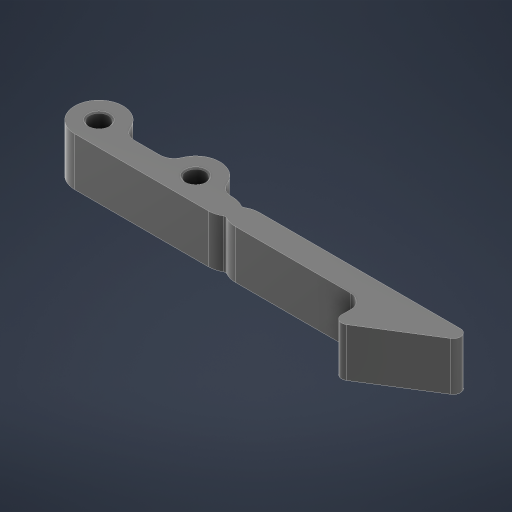
# Autodesk Inventor part: Battery_Clip
Saved by Autodesk Inventor 2024 (Build 280153000, 153)
## iProperties
Created: 2023-06-19
Part Number: Battery_Clip
Material: Nylon 6/6
Document SubType Name: Modeling
Designer: dzw04
Density: 1.13 g/cm^3
Appearance: Smooth - Black
Author: dzw04
Autodesk Inventor part; units mm, degrees
ref_plane "YZ Plane" through (0, 0, 0) normal (1, 0, 0) x (0, 1, 0)
ref_plane "XZ Plane" through (0, 0, 0) normal (0, 1, 0) x (-1, 0, 0)
ref_plane "XY Plane" through (0, 0, 0) normal (0, 0, 1) x (1, 0, 0)
sketch "Sketch1" plane through (0, 0, 0) normal (0, 1, 0) x (-1, 0, 0)
  circle A0 centre (0, 0) radius 2
  line L0 (-7.4162, 0) -> (-12.5838, 0) construction
  circle A1 centre (-20, 0) radius 2
  arc A2 (-4.6351, -1.875) -> (0, 5) centre (0, 0) ccw
  arc A3 (-24.6351, -1.875) -> (-15.3649, -1.875) centre (-20, 0) ccw
  line L1 (-5, 0) -> (-15, 0)
  arc A4 (-4.6351, -1.875) -> (-7.4162, 0) centre (-7.4162, -3) ccw
  arc A5 (-12.5838, 0) -> (-15.3649, -1.875) centre (-12.5838, -3) ccw
  line L2 (-27.4162, 0) -> (-74.7698, 0) construction
  line L3 (-80, 0) -> (-80, 12.5) construction
  line L4 (-80, 12.5) -> (-60, 12.5) construction
  line L5 (-75.5648, 2.772) -> (-62.295, 11.0656)
  line L6 (-80, 0) -> (-25, 0)
  line L7 (0, 5) -> (-57, 5)
  line L8 (-60, 8) -> (-60, 9.7936)
  arc A6 (-60, 8) -> (-57, 5) centre (-57, 8) ccw
  arc A7 (-60, 9.7936) -> (-62.295, 11.0656) centre (-61.5, 9.7936) ccw
  arc A8 (-75.5648, 2.772) -> (-74.7698, 0) centre (-74.7698, 1.5) ccw
  arc A9 (-24.6351, -1.875) -> (-27.4162, 0) centre (-27.4162, -3) ccw
  point P0 (-60, 5)
  point P1 (0, 5)
  point P2 (-74.7698, 0)
  point P3 (-7.4162, 0)
  point P4 (-27.4162, 0)
  dimension "d0" = 4
  dimension "d4" = 4
  dimension "d5" = 10
  dimension "d6" = 10
  dimension "d7" = 3
  dimension "d8" = 80
  dimension "d9" = 12.5
  dimension "d10" = 20
  dimension "d11" = 60
  dimension "d12" = 3
  dimension "d13" = 1.5
  dimension "d19" = 5
  dimension "d20" = 3
  constraints: 19 point on circle, 18 end point, 12 tangent, 11 point on line, 10 centre point, 4 horizontal, 3 coincident, 2 equal radius, 1 perpendicular, 1 vertical
  measures "d0" diameter of A0
  measures "d4" diameter of A1
  measures "d5" diameter of A2
  measures "d6" diameter of A3
  measures "d7" radius of A4
  measures "d8" distance of A2.centre L3.start
  measures "d9" distance of L3.start L3.end
  measures "d10" distance of L3.end L4.end
  measures "d11" distance of L7.start point (-60, 5)
  measures "d12" radius of A6
  measures "d13" radius of A7
  measures "d19" distance between parallel lines of L7 L2
  measures "d20" radius of A9
extrude "Extrusion1" add sketch "Sketch1" along normal blind 10
chamfer "Chamfer1" distance 0.25 angle 45 4 edges at (22, 10, 0) (2, 10, 0) (22, 0, 0) (2, 0, 0)
sketch "Sketch2" plane through (0, 10, 0) normal (0, 1, 0) x (1, 0, 0)
  circle A0 centre (20, 0) radius 2.25 projected
  arc A1 (75.5648, -2.772) -> (74.7698, 0) centre (74.7698, -1.5) ccw projected
  line L0 (74.7698, 0) -> (27.4162, 0) projected
  arc A2 (24.6351, 1.875) -> (27.4162, 0) centre (27.4162, 3) ccw projected
  arc A3 (24.6351, 1.875) -> (15.3649, 1.875) centre (20, 0) ccw projected
  arc A4 (12.5838, 0) -> (15.3649, 1.875) centre (12.5838, 3) ccw projected
  line L1 (12.5838, 0) -> (7.4162, 0) projected
  arc A5 (4.6351, 1.875) -> (7.4162, 0) centre (7.4162, 3) ccw projected
  arc A6 (4.6351, 1.875) -> (0, -5) centre (0, 0) ccw projected
  line L2 (0, -5) -> (57, -5) projected
  arc A7 (60, -8) -> (57, -5) centre (57, -8) ccw projected
  line L3 (60, -8) -> (60, -9.7936) projected
  arc A8 (60, -9.7936) -> (62.295, -11.0656) centre (61.5, -9.7936) ccw projected
  line L4 (62.295, -11.0656) -> (75.5648, -2.772) projected
  circle A9 centre (0, 0) radius 2.25 projected
sketch "Sketch3" plane through (0, 10, 0) normal (0, 1, 0) x (1, 0, 0)
  line L0 (27.4162, 0) -> (27.4162, -5) construction
  line L1 (0, -5) -> (57, -5) construction
  line L2 (27.4162, 0) -> (30.4162, 0) construction
  line L3 (30.4162, 0) -> (30.4162, -5) construction
  line L4 (30.4162, -5) -> (27.4162, -5) construction
  line L5 (27.4162, -5) -> (27.4162, 0) construction
  circle A0 centre (30.4162, -5) radius 0.75
  circle A1 centre (30.4162, 0) radius 0.75
  point P0 (0, 0)
  dimension "d21" = 3
  dimension "d22" = 5
  dimension "d23" = 1.5
  dimension "d24" = 1.5
  constraints: 10 end point, 2 centre point, 2 coincident, 2 parallel, 1 horizontal, 1 perpendicular, 1 point on line, 1 vertical
  measures "d21" distance of L3.end L4.end
  measures "d22" distance of L2.end L3.end
  measures "d23" diameter of A0
  measures "d24" diameter of A1
extrude "Extrusion2" cut sketch "Sketch3" against normal through all
fillet "Fillet1" radius 5 4 edges at (29.6662, 5, 5) (29.6662, 5, 0) (31.1662, 5, 0) (31.1662, 5, 5)
body "Solid1"
